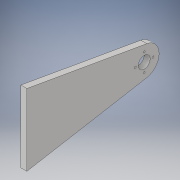
# Autodesk Inventor part: halter_seite
Saved by Autodesk Inventor 2017 (Build 210142000, 142)
## iProperties
Part Number: halter_seite
Material: Generisch
Document SubType Name: Modeling
Designer: Fabio
Density: 1 g/cm^3
Appearance: Vorgabe
Author: Fabio
Autodesk Inventor part; units mm, degrees
ref_plane "YZ Plane" through (0, 0, 0) normal (1, 0, 0) x (0, 1, 0)
ref_plane "XZ Plane" through (0, 0, 0) normal (0, 1, 0) x (-1, 0, 0)
ref_plane "XY Plane" through (0, 0, 0) normal (0, 0, 1) x (1, 0, 0)
sketch "Skizze1" plane through (0, 0, 0) normal (1, 0, 0) x (0, 1, 0)
  arc A0 (221.3076, 0) -> (200.6489, 24.6202) centre (196.3076, 0) ccw
  line L0 (196.3076, 0) -> (200.6489, 24.6202) construction
  line L1 (196.3076, 0) -> (221.3076, 0) construction
  line L2 (200.6489, 24.6202) -> (0, 60)
  line L3 (0, 60) -> (0, 0)
  arc A1 (200.6489, -24.6202) -> (221.3076, 0) centre (196.3076, 0) ccw
  line L4 (200.6489, -24.6202) -> (0, -60)
  line L5 (0, 0) -> (0, -60)
  dimension "d21" = 80
  dimension "d22" = 80
  dimension "d24" = 25
  dimension "d50" = 60
  dimension "d51" = 60
  constraints: 12 end point, 4 point on circle, 2 centre point, 2 symmetric about line, 2 vertical, 1 coincident, 1 other
  measures "d21" angle of L1 L0
  measures "d22" angle of L3 L2
  measures "d24" radius of A0
  measures "d50" distance of L2.end L3.end
  measures "d51" distance of L4.end L3.end
extrude "Extrusion1" add sketch "Skizze1" along normal blind 10
sketch "Skizze3" plane through (10, 0, 0) normal (1, 0, 0) x (0, 0, -1)
  arc A0 (24.6202, 200.6489) -> (-24.6202, 200.6489) centre (0, 196.3076) ccw projected
  point P0 (0, 0)
  constraints: 1 coincident
hole "Bohrung2" at (10, 196.3076, 0) direction (-1, 0, 0) diameter 20 end through all
sketch "Skizze4" plane through (10, 0, 0) normal (1, 0, 0) x (0, 0, -1)
  arc A0 (24.6202, 200.6489) -> (-24.6202, 200.6489) centre (0, 196.3076) ccw projected
  line L0 (60, 0) -> (24.6202, 200.6489) projected
  line L1 (0, 0) -> (0, 181.3076) construction
  point P0 (15, 196.3076)
  point P1 (0, 211.3076)
  point P2 (-15, 196.3076)
  dimension "d34" = 15
  dimension "d38" = 360
  constraints: 2 end point, 1 vertical, 5 other
  measures "d34" distance of L1.end A0.centre
hole "Bohrung3" at (10, 181.3076, 0) at (10, 196.3076, -15) at (10, 211.3076, 0) at (10, 196.3076, 15) direction (-1, 0, 0) diameter 3 end through all
